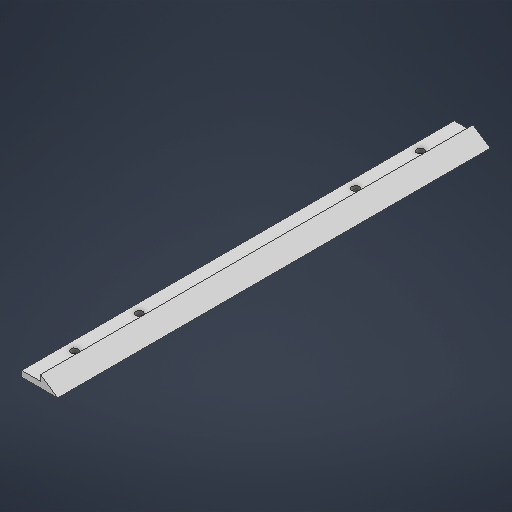
# Autodesk Inventor part: pługmoj
Saved by Autodesk Inventor 2026.2 (Build 302298010, 298A)
## iProperties
Created: 2026-05-09
Part Number: pługmoj
Material: Ogólny
Document SubType Name: Modeling
Designer: karol
Density: 1 g/cm^3
Appearance: Domyślna
Author: karol
Autodesk Inventor part; units mm, degrees
ref_plane "YZ Plane" through (0, 0, 0) normal (1, 0, 0) x (0, 1, 0)
ref_plane "XZ Plane" through (0, 0, 0) normal (0, 1, 0) x (-1, 0, 0)
ref_plane "XY Plane" through (0, 0, 0) normal (0, 0, 1) x (1, 0, 0)
sketch "Szkic1" plane through (0, 0, 0) normal (0, 1, 0) x (-1, 0, 0)
  line L0 (0, 0) -> (6.5, 0)
  line L1 (6.5, 0) -> (6.5, -150)
  line L2 (6.5, -150) -> (0, -150)
  line L3 (0, -150) -> (0, 0)
  dimension "d0" = 6.5
  dimension "d1" = 150
  constraints: 8 end point, 2 parallel, 1 horizontal, 1 perpendicular
  measures "d0" distance of L1.end L2.end
  measures "d1" distance of L0.end L1.end
extrude "Wyciągnięcie proste1" add sketch "Szkic1" along normal blind 2
sketch "Szkic8" plane through (-6.5, 0, 0) normal (0, 0, 1) x (1, 0, 0)
  line L0 (6.5, 2) -> (0, 2) projected
  line L1 (6.5, 2) -> (12.5, 2)
  line L2 (12.5, 2) -> (12.5, -2)
  line L3 (12.5, -2) -> (6.5, -2)
  line L4 (6.5, -2) -> (6.5, 2)
  line L5 (12.5, -2) -> (6.5, 2)
  point P0 (6.5, 0)
  dimension "d34" = 6
  dimension "d35" = 4
  constraints: 10 end point, 2 parallel, 1 horizontal, 1 perpendicular
  measures "d34" distance of L2.end L3.end
  measures "d35" distance of L1.end L2.end
extrude "Wyciągnięcie proste6" add sketch "Szkic8" against normal blind 150 contours L5 L3 L4
sketch "Szkic9" plane through (0, 0, -150) normal (-1, 0, 0) x (0, 0, 1)
  line L0 (0, 2) -> (0, -2) projected
  line L1 (0, -2) -> (150, -2)
  line L2 (150, -2) -> (150, 0)
  line L3 (150, 0) -> (0, 0)
  line L4 (0, 0) -> (0, -2)
  line L5 (0, 2) -> (150, 2) projected
  line L6 (150, 0) -> (0, 0)
  line L7 (0, 0) -> (0, 2)
  line L8 (0, 2) -> (150, 2)
  line L9 (150, 2) -> (150, 0)
  constraints: 16 end point, 4 parallel, 2 horizontal, 2 perpendicular
extrude "Wyciągnięcie proste7" cut sketch "Szkic9" along normal blind 10 contours L5 L9 L3 L0
extrude "Wyciągnięcie proste8" add sketch "Szkic9" along normal blind 6.5 contours L3 L2 L1 L0
sketch "Szkic10" plane through (0, 0, 0) normal (0, 1, 0) x (1, 0, 0)
  circle A0 centre (-3.25, 15) radius 1.25
  line L0 (0, 0) -> (-6.5, 0) projected
  line L1 (-6.5, 0) -> (-6.5, 150) projected
  circle A1 centre (-3.25, 37.5) radius 1.25
  circle A2 centre (-3.25, 112.5) radius 1.25
  circle A3 centre (-3.25, 135) radius 1.25
  line L2 (0, 150) -> (-6.5, 150) projected
  point P0 (-3.25, 0)
  point P1 (-3.25, 150)
  dimension "d42" = 2.5
  dimension "d43" = 15
  dimension "d44" = 3.25
  dimension "d45" = 2.5
  dimension "d46" = 3.25
  dimension "d47" = 37.5
  dimension "d49" = 2.5
  dimension "d50" = 2.5
  dimension "d53" = 15
  dimension "d54" = 37.5
  dimension "d55" = 3.25
  dimension "d56" = 3.25
  constraints: 4 centre point, 2 midpoint
  measures "d42" diameter of A0
  measures "d43" distance of point (-3.25, 0) A0.centre
  measures "d44" distance from line of L1 A0.centre
  measures "d45" diameter of A1
  measures "d46" distance from line of L1 A1.centre
  measures "d47" distance from line of L0 A1.centre
  measures "d49" diameter of A2
  measures "d50" diameter of A3
  measures "d53" distance of point (-3.25, 150) A3.centre
  measures "d54" distance from line of L2 A2.centre
  measures "d55" distance from line of L1 A2.centre
  measures "d56" distance from line of L1 A3.centre
extrude "Wyciągnięcie proste9" cut sketch "Szkic10" against normal blind 2
thread "Gwint5" size "M3x0.5" class "6H" standard "ANSI Metric M Profile" full length
thread "Gwint6" size "M3x0.5" class "6H" standard "ANSI Metric M Profile" full length
thread "Gwint8" size "M3x0.5" class "6H" standard "ANSI Metric M Profile" full length
thread "Gwint9" size "M3x0.5" class "6H" standard "ANSI Metric M Profile" full length
